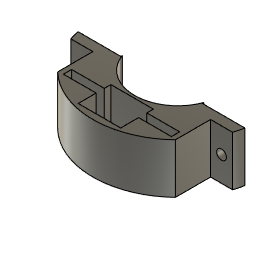
Housing_v3_part2 (Autodesk Fusion 360 design; units mm, degrees)
Autodesk Fusion 360 part; units mm, degrees
note: some values were not read from the file. Set by a fixed rule: which sketch regions a step uses.
sketch "Sketch1" plane through (0, 0, 0) normal (0, 0, 1) x (1, 0, 0)
  circle A0 centre (0, 0) radius 26
  circle A1 centre (0, 0) radius 13.25
  line L0 (0.2027, -25.9992) -> (0.2027, -4.4992)
  line L1 (0.2027, -4.4992) -> (-25.6078, -4.4992)
  line L2 (0.2027, -4.4992) -> (25.6078, -4.4992)
  dimension "d1" = 52
  dimension "d2" = 26.5
  dimension "d3" = 21.5
  constraint coincident A0.centre A1.centre
  constraint coincident A0 L0.start
  constraint vertical L0
  constraint coincident A0 L1.end
  constraint perpendicular L0 L1
  constraint coincident A0 L2.end
  constraint perpendicular L0 L2
  measures "d1" diameter of A0
  measures "d2" diameter of A1
  measures "d3" distance of L0.start L0.end
extrude "Extrude1" add sketch "Sketch1" along normal blind 15.25 contours A0 A1 L0 L1 | A0 A1 L0 L2
ref_plane "WorkPlane1" through (0, -26, 8.3665) normal (0, -1, 0) x (-1, 0, 0)
sketch "Sketch4" plane through (0, -26, 8.3665) normal (0, -1, 0) x (1, 0, 0)
  spline S0 degree 3 poles (-20.8578, -0.7415) (-20.8578, -0.818) (-20.8649, -0.8948) (-20.8924, -1.0435) (-20.9128, -1.1154) (-20.9889, -1.3172) (-21.0602, -1.4332) (-21.2709, -1.6961) (-21.4384, -1.8135) (-21.7794, -1.9619) (-21.953, -1.9915) (-22.2831, -1.9915) (-22.468, -1.9536) (-22.8127, -1.7912) (-22.9729, -1.6694) (-23.1674, -1.413) (-23.2314, -1.3059) (-23.3026, -1.1148) (-23.3223, -1.0462) (-23.3499, -0.9001) (-23.3578, -0.8227) (-23.3578, -0.6603) (-23.3499, -0.5829) (-23.3223, -0.4369) (-23.3026, -0.3683) (-23.2314, -0.1772) (-23.1674, -0.0701) (-22.9729, 0.1863) (-22.8127, 0.3081) (-22.468, 0.4705) (-22.2831, 0.5085) (-21.953, 0.5085) (-21.7794, 0.4788) (-21.4384, 0.3304) (-21.2709, 0.2131) (-21.0602, -0.0498) (-20.9889, -0.1658) (-20.9128, -0.3677) (-20.8924, -0.4395) (-20.8649, -0.5882) (-20.8578, -0.665) (-20.8578, -0.7415) knots 0 0 0 0 0.022956 0.022956 0.045913 0.045913 0.091826 0.091826 0.180047 0.180047 0.268267 0.268267 0.368193 0.368193 0.468118 0.468118 0.516845 0.516845 0.541208 0.541208 0.565572 0.565572 0.589935 0.589935 0.614298 0.614298 0.663025 0.663025 0.76295 0.76295 0.862876 0.862876 0.951096 0.951096 1.039317 1.039317 1.08523 1.08523 1.108187 1.108187 1.131143 1.131143 1.131143 1.131143
  spline S1 degree 3 poles (23.3578, -0.7415) (23.3578, -0.8227) (23.3499, -0.9001) (23.3223, -1.0462) (23.3026, -1.1148) (23.2314, -1.3059) (23.1674, -1.413) (22.9729, -1.6694) (22.8127, -1.7912) (22.468, -1.9536) (22.2831, -1.9915) (21.953, -1.9915) (21.7794, -1.9619) (21.4384, -1.8135) (21.2709, -1.6961) (21.0602, -1.4332) (20.9889, -1.3172) (20.9128, -1.1154) (20.8924, -1.0435) (20.8649, -0.8948) (20.8578, -0.818) (20.8578, -0.665) (20.8649, -0.5882) (20.8924, -0.4395) (20.9128, -0.3677) (20.9889, -0.1658) (21.0602, -0.0498) (21.2709, 0.2131) (21.4384, 0.3304) (21.7794, 0.4788) (21.953, 0.5085) (22.2831, 0.5085) (22.468, 0.4705) (22.8127, 0.3081) (22.9729, 0.1863) (23.1674, -0.0701) (23.2314, -0.1772) (23.3026, -0.3683) (23.3223, -0.4369) (23.3499, -0.5829) (23.3578, -0.6603) (23.3578, -0.7415) knots 0 0 0 0 0.024363 0.024363 0.048727 0.048727 0.097454 0.097454 0.197379 0.197379 0.297304 0.297304 0.385525 0.385525 0.473746 0.473746 0.519659 0.519659 0.542615 0.542615 0.565572 0.565572 0.588528 0.588528 0.611485 0.611485 0.657398 0.657398 0.745618 0.745618 0.833839 0.833839 0.933764 0.933764 1.03369 1.03369 1.082416 1.082416 1.10678 1.10678 1.131143 1.131143 1.131143 1.131143
  line L0 (-22, -1) -> (-18, -1)
  line L1 (22, -1) -> (18, -1)
  line L2 (-18, 8.8173) -> (-28, 8.8173)
  line L3 (-28, 8.8173) -> (-28, -12)
  line L4 (-28, -12) -> (-18, -12)
  line L5 (-18, -12) -> (-18, 8.8173)
  line L6 (18, 8.8173) -> (29, 8.8173)
  line L7 (29, 8.8173) -> (29, -13)
  line L8 (29, -13) -> (18, -13)
  line L9 (18, -13) -> (18, 8.8173)
  dimension "d15" = 4
  dimension "d16" = 4
  constraint horizontal L0
  constraint horizontal L1
  constraint horizontal L2
  constraint vertical L3
  constraint horizontal L4
  constraint vertical L5
  constraint horizontal L6
  constraint vertical L7
  constraint horizontal L8
  constraint vertical L9
  measures "d15" distance of L0.start L0.end
  measures "d16" distance of L1.start L1.end
extrude "Extrude4" cut sketch "Sketch4" against normal blind 18 contours S0 | S1 | L2 L3 L4 L5 | L6 L7 L8 L9
sketch "Sketch5" plane through (0, 0, 15.25) normal (0, 0, 1) x (-1, 0, 0)
  line L0 (18, 8) -> (18, 18.7617)
  arc A0 (18, 18.7617) -> (-18, 18.7617) centre (0, 0) ccw
  line L1 (-18, 18.7617) -> (-18, 8)
  line L2 (-18, 8) -> (-24.7386, 8)
  arc A1 (-24.7386, 8) -> (-25.6078, 4.4992) centre (0, 0) ccw
  line L3 (-25.6078, 4.4992) -> (-12.4627, 4.4992)
  arc A2 (12.4627, 4.4992) -> (-12.4627, 4.4992) centre (0, 0) ccw
  line L4 (12.4627, 4.4992) -> (25.6078, 4.4992)
  arc A3 (25.6078, 4.4992) -> (24.7386, 8) centre (0, 0) ccw
  line L5 (24.7386, 8) -> (18, 8)
  line L6 (0, 16) -> (-16.5, 16)
  line L7 (0, 16) -> (16.5, 16)
  line L8 (16.5, 16) -> (-16.5327, 16)
  line L9 (-16.5327, 16) -> (-16.5327, 18.5)
  line L10 (-16.5327, 18.5) -> (16.5, 18.5)
  line L11 (16.5, 18.5) -> (16.5, 16)
  line L12 (0, 16) -> (-6.5, 16)
  line L13 (-6.5, 16) -> (6.5, 16)
  line L14 (6.5, 16) -> (6.5, 23)
  line L15 (6.5, 23) -> (-6.5, 23)
  line L16 (-6.5, 23) -> (-6.5, 16)
  line L17 (6.5, 16) -> (-6.5, 16)
  line L18 (-6.5, 16) -> (-6.5, 14)
  line L19 (-6.5, 14) -> (6.5, 14)
  line L20 (6.5, 14) -> (6.5, 16)
  dimension "d19" = 16.5
  dimension "d20" = 16.5
  dimension "d21" = 2.5
  dimension "d22" = 6.5
  dimension "d23" = 13
  dimension "d24" = 7
  dimension "d25" = 2
  constraint perpendicular L1 L6
  constraint parallel L6 L7
  constraint horizontal L8
  constraint vertical L9
  constraint horizontal L10
  constraint vertical L11
  constraint coincident L6 L12.end
  constraint horizontal L13
  constraint vertical L14
  constraint horizontal L15
  constraint vertical L16
  constraint horizontal L17
  constraint vertical L18
  constraint horizontal L19
  constraint vertical L20
  measures "d19" distance of L6.start L6.end
  measures "d20" distance of L6.start L7.end
  measures "d21" distance of L7.end L10.end
  measures "d22" distance of L6.start L12.end
  measures "d23" distance of L12.end L13.end
  measures "d24" distance of L12.end L15.end
  measures "d25" distance of L13.end L19.end
extrude "Extrude5" cut sketch "Sketch5" against normal blind 13 contours L6 L7 L8 L12 L13 L17 L18 L19 L20 | L6 L7 L8 L10 L12 L13 L14 L16 L17 | L6 L8 L9 L10 L16 | L7 L8 L10 L11 L14 | L10 L14 L15 L16
sketch "Sketch6" plane through (0, -8, 0) normal (0, -1, 0) x (1, 0, 0)
  line L0 (-18, 15.25) -> (-24.7386, 15.25)
  line L1 (-24.7386, 15.25) -> (-24.7386, 0)
  line L2 (-24.7386, 0) -> (-18, 0)
  line L3 (-18, 0) -> (-18, 15.25)
  circle A0 centre (-21.3693, 7.625) radius 1.5
  dimension "d28" = 3
  measures "d28" diameter of A0
extrude "Extrude6" cut sketch "Sketch6" against normal blind 37 contours A0
sketch "Sketch7" plane through (0, -8, 0) normal (0, -1, 0) x (1, 0, 0)
  line L0 (18, 0) -> (24.7386, 0)
  line L1 (24.7386, 0) -> (24.7386, 15.25)
  line L2 (24.7386, 15.25) -> (18, 15.25)
  line L3 (18, 15.25) -> (18, 0)
  circle A0 centre (21.3693, 7.625) radius 1.5
  dimension "d31" = 3
  measures "d31" diameter of A0
extrude "Extrude7" cut sketch "Sketch7" against normal blind 41 contours A0
extrude "Extrude8" cut 1 faces at (-2.1667, -23, 10.9167) along direction (0, -1, 0) blind 1
extrude "Extrude9" cut 1 faces at (2.1667, -22.1667, 2.25) along direction (0, 0, -1) blind 1
extrude "Extrude10" cut 2 faces at (14.9316, -4.4992, 7.625) (-14.9316, -4.4992, 7.625) along direction (0, -1, 0) blind 0.5
